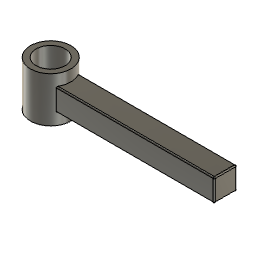
Infrared Sensor Mount Attempt 1- Sam v3 (Autodesk Fusion 360 design; units mm, degrees)
Autodesk Fusion 360 part; units mm, degrees
note: some values were not read from the file. Set by a fixed rule: which sketch regions a step uses.
sketch "Sketch1" plane through (0, 0, 0) normal (0, 0, 1) x (1, 0, 0)
  circle A0 centre (0, 0) radius 6.45
  circle A1 centre (0, 0) radius 6.35
  circle A2 centre (0, 0) radius 8.95
  line L0 (0, 0) -> (0, 5)
  line L1 (0, 5) -> (7.4231, 5)
  line L2 (7.4231, 5) -> (77.4231, 5)
  line L3 (77.4231, 5) -> (77.4231, -5)
  line L4 (77.4231, -5) -> (7.4231, -5)
  line L5 (7.4231, -5) -> (7.4231, 5)
  dimension "d1" = 12.9
  dimension "d2" = 12.7
  dimension "d3" = 17.9
  dimension "d4" = 5
  dimension "d5" = 70
  dimension "d6" = 10
  constraint coincident A0.centre A1.centre
  constraint concentric A0 A2
  constraint vertical L0
  constraint coincident A2 L1.end
  constraint perpendicular L0 L1
  constraint horizontal L2
  constraint vertical L3
  constraint horizontal L4
  constraint vertical L5
  measures "d1" diameter of A0
  measures "d2" diameter of A1
  measures "d3" diameter of A2
  measures "d4" distance of A0.centre L0.end
  measures "d5" distance of L1.end L2.end
  measures "d6" distance of L1.end L4.end
extrude "Extrude2" add sketch "Sketch1" along normal blind 10 and the other way blind 10 contours A2 L5 | A2 L5
extrude "Extrude3" add sketch "Sketch1" along normal blind 5 and the other way blind 5 contours A2 L2 L3 L4
fillet "Fillet1" radius 0.5 4 edges at (42.4231, -5, 5) (42.4231, -5, -5) (42.4231, 5, -5) (42.4231, 5, 5) 1 faces at (77.4231, 1.6667, -1.6667)
named bodies: "AS Flag (Sam)"
